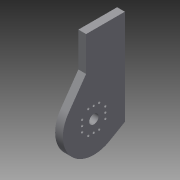
# Autodesk Inventor part: cadera
Saved by Autodesk Inventor 2015 (Build 190159000, 159)
## iProperties
Created: 2015-08-01
Part Number: cadera
Material: Genérico
Document SubType Name: Modeling
Designer: Roberto
Density: 1 g/cm^3
Appearance: Valor por defecto
Author: Roberto
Autodesk Inventor part; units mm, degrees
ref_plane "YZ Plane" through (0, 0, 0) normal (1, 0, 0) x (0, 1, 0)
ref_plane "XZ Plane" through (0, 0, 0) normal (0, 1, 0) x (-1, 0, 0)
ref_plane "XY Plane" through (0, 0, 0) normal (0, 0, 1) x (1, 0, 0)
ref_plane "Plano de trabajo1" through (129.4922, 102.1402, -54.3752) normal (1, 0, 0) x (0, 1, 0)
sketch "Boceto1" plane through (129.4922, 102.1402, -54.3752) normal (1, 0, 0) x (0, 1, 0)
  circle A0 centre (-7.5, 0) radius 0.75 projected
  circle A1 centre (3.5, 7.5) radius 0.75 projected
  circle A2 centre (-3.5, 7.5) radius 0.75 projected
  circle A3 centre (7.5, 0) radius 0.75 projected
  circle A4 centre (-3.5, -7.5) radius 0.75 projected
  circle A5 centre (0, -7.5) radius 0.75 projected
  circle A6 centre (3.5, -7.5) radius 0.75 projected
  circle A7 centre (7.5, 3.5) radius 0.75 projected
  circle A8 centre (7.5, -3.5) radius 0.75 projected
  circle A9 centre (0, 7.5) radius 0.75 projected
  circle A10 centre (-7.5, -3.5) radius 0.75 projected
  circle A11 centre (-7.5, 3.5) radius 0.75 projected
  circle A12 centre (0, 0) radius 3 projected
  circle A13 centre (0, 0) radius 10.5 projected
  arc A14 (-16.383, 11.4715) -> (10, -17.3205) centre (0, 0) ccw
  line L0 (-16.383, 11.4715) -> (-10, 20.5875)
  line L1 (-10, 20.5875) -> (-10, 45)
  line L2 (-10, 45) -> (15, 45)
  line L3 (15, 45) -> (15, -14.4338)
  line L4 (15, -14.4338) -> (10, -17.3205)
  point P0 (-102.1402, 54.3752)
  dimension "d0" = 20
  dimension "d1" = 45
  dimension "d2" = 10
  dimension "d3" = 25
  dimension "d4" = 145
  dimension "d5" = 60
  constraints: 10 end point, 3 point on circle, 2 perpendicular, 2 tangent, 1 centre point, 1 coincident, 1 vertical
  measures "d0" radius of A14
  measures "d1" distance from line of A12.centre L2
  measures "d2" distance from line of A12.centre L1
  measures "d3" distance of L1.end L2.end
  measures "d4" angle of L1 L0
  measures "d5" angle of L4 L3
extrude "Extrusión1" add sketch "Boceto1" along normal blind 5 contours A13 | L0 L1 L2 L3 L4 A14
